Autodesk Inventor part; units mm, degrees
(part 5 of 7)
sketch "Dach z grawerem" plane through (0, 0, 2) normal (0, 0, 1) x (1, 0, 0)
  line L0 (-37.1273, -35.5639) -> (-39.2128, -35.5639) projected
  line L1 (-39.2128, -35.5639) -> (-40.0969, -34.6798) projected
  line L2 (-40.0969, -34.6798) -> (-40.0969, -31.5163) projected
  line L3 (-40.0969, -31.5163) -> (-39.2128, -30.6321) projected
  line L4 (-39.2128, -30.6321) -> (-37.1273, -30.6321) projected
  line L5 (-37.1273, -30.6321) -> (-36.2431, -31.5163) projected
  line L6 (-36.2431, -31.5163) -> (-36.2431, -34.6798) projected
  line L7 (-36.2431, -34.6798) -> (-37.1273, -35.5639) projected
  line L8 (-36.2431, -25.5358) -> (-40.0763, -25.5358) projected
  line L9 (-40.0763, -25.5358) -> (-40.7431, -24.2816) projected
  line L10 (-40.7431, -24.2816) -> (-36.2431, -24.2816) projected
  line L11 (-36.2431, -24.2816) -> (-36.2431, -25.5358) projected
  line L12 (-37.1273, -23.6971) -> (-39.2128, -23.6971) projected
  line L13 (-39.2128, -23.6971) -> (-40.0969, -22.8129) projected
  line L14 (-40.0969, -22.8129) -> (-40.0969, -19.6494) projected
  line L15 (-40.0969, -19.6494) -> (-39.2128, -18.7653) projected
  line L16 (-39.2128, -18.7653) -> (-37.1273, -18.7653) projected
  line L17 (-37.1273, -18.7653) -> (-36.2431, -19.6494) projected
  line L18 (-36.2431, -19.6494) -> (-36.2431, -22.8129) projected
  line L19 (-36.2431, -22.8129) -> (-37.1273, -23.6971) projected
  line L20 (4.635, -37.5613) -> (4.635, -40.3224) projected
  line L21 (4.635, -40.3224) -> (3.9927, -39.8015) projected
  line L22 (3.9927, -39.8015) -> (3.9927, -38.323) projected
  line L23 (3.9927, -38.323) -> (3.6441, -38.323) projected
  line L24 (3.6441, -38.323) -> (3.6441, -39.9973) projected
  line L25 (3.6441, -39.9973) -> (3.0527, -39.5176) projected
  line L26 (3.0527, -39.5176) -> (3.0527, -38.323) projected
  line L27 (3.0527, -38.323) -> (2.7042, -38.323) projected
  line L28 (2.7042, -38.323) -> (2.7042, -40.2441) projected
  line L29 (2.7042, -40.2441) -> (2.0619, -39.7193) projected
  line L30 (2.0619, -39.7193) -> (2.0619, -37.5613) projected
  line L31 (2.0619, -37.5613) -> (4.635, -37.5613) projected
  line L32 (4.635, -25.0404) -> (4.635, -27.8015) projected
  line L33 (4.635, -27.8015) -> (3.9927, -27.2806) projected
  line L34 (3.9927, -27.2806) -> (3.9927, -25.8022) projected
  line L35 (3.9927, -25.8022) -> (3.6421, -25.8022) projected
  line L36 (3.6421, -25.8022) -> (3.6421, -27.4764) projected
  line L37 (3.6421, -27.4764) -> (3.0508, -26.9967) projected
  line L38 (3.0508, -26.9967) -> (3.0508, -25.8022) projected
  line L39 (3.0508, -25.8022) -> (2.0795, -25.8022) projected
  line L40 (2.0795, -25.8022) -> (1.635, -25.0404) projected
  line L41 (1.635, -25.0404) -> (4.635, -25.0404) projected
  line L42 (3.8791, -22.7395) -> (3.2368, -22.7395) projected
  line L43 (3.2368, -22.7395) -> (3.2368, -22.1559) projected
  line L44 (3.2368, -22.1559) -> (3.8791, -22.1559) projected
  line L45 (3.8791, -22.1559) -> (3.8791, -22.7395) projected
  line L46 (5.0697, -18.5097) -> (2.6572, -18.5097) projected
  line L47 (2.6572, -18.5097) -> (2.0658, -17.9771) projected
  line L48 (2.0658, -17.9771) -> (2.0658, -16.2421) projected
  line L49 (2.0658, -16.2421) -> (2.6572, -15.7095) projected
  line L50 (2.6572, -15.7095) -> (4.6408, -15.7095) projected
  line L51 (2.7022, -16.4712) -> (2.7022, -17.7441) projected
  line L52 (2.7022, -17.7441) -> (4.6134, -17.7441) projected
  line L53 (4.6134, -17.7441) -> (5.0697, -18.5097) projected
  line L54 (4.635, -10.6279) -> (4.635, -12.8563) projected
  line L55 (2.7042, -12.778) -> (2.0619, -12.2532) projected
  line L56 (2.0619, -12.2532) -> (2.0619, -10.6259) projected
  line L57 (2.0619, -10.6259) -> (2.6454, -10.0952) projected
  line L58 (2.6454, -10.0952) -> (4.0416, -10.0952) projected
  line L59 (4.0416, -10.0952) -> (4.635, -10.6279) projected
  line L60 (2.7042, -4.949) -> (2.7042, -6.87) projected
  line L61 (2.7042, -6.87) -> (2.0619, -6.3452) projected
  line L62 (2.0619, -6.3452) -> (2.0619, -4.7179) projected
  line L63 (2.0619, -4.7179) -> (2.6454, -4.1873) projected
  line L64 (2.6454, -4.1873) -> (4.0416, -4.1873) projected
  line L65 (4.0514, -3.8191) -> (1.635, -3.8191) projected
  line L66 (1.635, -3.8191) -> (2.0795, -3.0535) projected
  line L67 (2.0795, -3.0535) -> (2.7786, -3.0535) projected
  line L68 (2.7786, -3.0535) -> (2.7786, -1.7806) projected
  line L69 (2.7786, -1.7806) -> (2.0619, -1.7806) projected
  line L70 (2.0619, -1.7806) -> (2.0658, -1.0189) projected
  line L71 (2.0658, -1.0189) -> (4.0514, -1.0189) projected
  line L72 (-58.6053, 8.1191) -> (-59.4082, 7.5578) projected
  line L73 (-59.4082, 7.5578) -> (-60.7496, 8.4879) projected
  line L74 (-60.7496, 8.4879) -> (-60.7496, 12.7634) projected
  line L75 (-60.7496, 12.7634) -> (-56.4611, 12.7634) projected
  line L76 (-59.4571, 13.4129) -> (-61.4611, 13.4129) projected
  line L77 (-61.4611, 13.4129) -> (-60.7137, 14.7445) projected
  line L78 (-60.7137, 14.7445) -> (-59.6889, 14.7445) projected
  line L79 (-59.6889, 14.7445) -> (-59.3592, 15.0676) projected
  line L80 (-59.3592, 15.0676) -> (-59.3592, 17.2347) projected
  line L81 (-59.3592, 17.2347) -> (-60.743, 17.2347) projected
  line L82 (-60.743, 17.2347) -> (-60.743, 18.5663) projected
  line L83 (-60.743, 18.5663) -> (-56.4611, 18.5663) projected
  line L84 (-56.4611, 18.5663) -> (-56.4611, 14.343) projected
  line L85 (-56.4611, 14.343) -> (-57.8057, 13.4129) projected
  line L86 (-57.8057, 13.4129) -> (-58.762, 14.095) projected
  line L87 (-58.762, 14.095) -> (-59.4571, 13.4129) projected
  line L88 (-56.4611, 29.8554) -> (-56.4611, 24.4344) projected
  line L89 (-56.4611, 24.4344) -> (-57.5218, 25.3515) projected
  line L90 (-57.5218, 25.3515) -> (-57.5218, 26.4807) projected
  line L91 (-57.5218, 26.4807) -> (-60.7137, 26.4807) projected
  line L92 (-60.7137, 26.4807) -> (-61.4611, 27.8123) projected
  line L93 (-61.4611, 27.8123) -> (-57.5218, 27.8123) projected
  line L94 (-57.5218, 27.8123) -> (-57.5218, 28.9416) projected
  line L95 (-57.5218, 28.9416) -> (-56.4611, 29.8554) projected
  line L96 (-75.6403, -50.5982) -> (-75.4415, -50.7741) projected
  line L97 (-75.4415, -50.7741) -> (-75.2314, -50.5982) projected
  line L98 (-75.2314, -50.5982) -> (-75.2314, -48.4484) projected
  line L99 (-75.2314, -48.4484) -> (-74.3267, -47.8041) projected
  line L100 (-74.3267, -47.8041) -> (-73.3854, -48.4689) projected
  line L101 (-73.3854, -48.4689) -> (-73.3854, -51.8113) projected
  line L102 (-73.3854, -51.8113) -> (-74.1279, -51.151) projected
  line L103 (-74.1279, -51.151) -> (-74.1279, -49.0149) projected
  line L104 (-74.1279, -49.0149) -> (-74.3267, -48.8367) projected
  line L105 (-74.3267, -48.8367) -> (-74.5368, -49.0149) projected
  line L106 (-74.5368, -49.0149) -> (-74.5368, -51.1648) projected
  line L107 (-75.6403, -41.3616) -> (-75.6403, -43.7787) projected
  line L108 (-75.6403, -43.7787) -> (-76.3874, -43.1184) projected
  line L109 (-76.3874, -43.1184) -> (-76.3874, -40.4112) projected
  line L110 (-76.3874, -40.4112) -> (-73.4082, -40.4112) projected
  line L111 (-72.8782, -41.3616) -> (-75.6403, -41.3616) projected
  line L112 (-73.3854, -39.4905) -> (-74.3267, -40.1553) projected
  line L113 (-74.3267, -40.1553) -> (-75.4141, -39.3854) projected
  line L114 (-75.4141, -39.3854) -> (-75.4141, -37.4229) projected
  line L115 (-75.4141, -37.4229) -> (-76.8854, -37.4229) projected
  line L116 (-76.8854, -37.4229) -> (-76.3622, -36.4725) projected
  line L117 (-76.3622, -36.4725) -> (-73.3854, -36.4725) projected
  line L118 (-73.3854, -36.4725) -> (-73.3854, -39.4905) projected
  line L119 (-74.5368, -28.9836) -> (-75.4438, -29.6302) projected
  line L120 (-75.4438, -29.6302) -> (-76.3828, -28.9653) projected
  line L121 (-76.3828, -28.9653) -> (-76.3828, -25.623) projected
  line L122 (-76.3828, -25.623) -> (-75.6403, -26.2764) projected
  line L123 (-75.6403, -26.2764) -> (-75.6403, -28.417) projected
  line L124 (-75.6403, -28.417) -> (-75.4415, -28.593) projected
  line L125 (-75.4415, -28.593) -> (-75.2314, -28.417) projected
  line L126 (-75.2314, -28.417) -> (-75.2314, -26.2672) projected
  line L127 (-75.2314, -26.2672) -> (-74.3267, -25.623) projected
  line L128 (-74.3267, -25.623) -> (-73.3854, -26.2878) projected
  line L129 (-73.3854, -26.2878) -> (-73.3854, -29.6302) projected
  line L130 (-73.3854, -29.6302) -> (-74.1279, -28.9699) projected
  line L131 (-74.1279, -28.9699) -> (-74.1279, -26.8338) projected
  line L132 (-74.1279, -26.8338) -> (-74.3267, -26.6556) projected
  line L133 (-74.3267, -26.6556) -> (-74.5368, -26.8338) projected
  line L134 (-74.5368, -26.8338) -> (-74.5368, -28.9836) projected
  line L135 (-75.6403, -19.1804) -> (-75.6403, -21.5975) projected
  line L136 (-75.6403, -21.5975) -> (-76.3874, -20.9373) projected
  line L137 (-76.3874, -20.9373) -> (-76.3874, -18.23) projected
  line L138 (-76.3874, -18.23) -> (-73.4082, -18.23) projected
  line L139 (-73.4082, -18.23) -> (-72.8782, -19.1804) projected
  line L140 (-72.8782, -19.1804) -> (-75.6403, -19.1804) projected
  line L141 (-73.3854, -17.3093) -> (-74.3267, -17.9742) projected
  line L142 (-74.3267, -17.9742) -> (-75.4141, -17.2042) projected
  line L143 (-75.4141, -17.2042) -> (-75.4141, -15.2418) projected
  line L144 (-75.4141, -15.2418) -> (-76.8854, -15.2418) projected
  line L145 (-76.8854, -15.2418) -> (-76.3622, -14.2914) projected
  line L146 (-62.0137, -37.4249) -> (-62.0137, -39.8107) projected
  line L147 (-62.0137, -39.8107) -> (-63.3037, -39.2171) projected
  line L148 (-63.3037, -39.2171) -> (-71.4886, -39.2171) projected
  line L149 (-71.4886, -39.2171) -> (-71.4886, -37.4934) projected
  line L150 (-71.4886, -37.4934) -> (-63.6576, -37.4934) projected
  line L151 (-63.6576, -37.4934) -> (-63.6576, -36.66) projected
  line L152 (-63.6576, -36.66) -> (-62.0137, -37.4249) projected
  line L153 (-69.8448, -24.845) -> (-69.8448, -28.7491) projected
  line L154 (-69.8448, -28.7491) -> (-71.4886, -27.9728) projected
  line L155 (-71.4886, -27.9728) -> (-71.4886, -23.1212) projected
  line L156 (-71.4886, -23.1212) -> (-63.5891, -23.1212) projected
  line L157 (-63.5891, -23.1212) -> (-63.0069, -22.4705) projected
  line L158 (-62.0137, -10.5642) -> (-62.0137, -12.95) projected
  line L159 (-62.0137, -12.95) -> (-63.3037, -12.3564) projected
  line L160 (-63.3037, -12.3564) -> (-71.7398, -12.3564) projected
  line L161 (-71.7398, -12.3564) -> (-64.7078, -7.0938) projected
  line L162 (-64.7078, -7.0938) -> (-69.8448, -7.0938) projected
  line L163 (-69.8448, -7.0938) -> (-69.8448, -9.4911) projected
  line L164 (-69.8448, -9.4911) -> (-71.4886, -8.7263) projected
  line L165 (-71.4886, -8.7263) -> (-71.4886, -5.8381) projected
  line L166 (-71.4886, -5.8381) -> (-70.0731, -6.4888) projected
  line L167 (-70.0731, -6.4888) -> (-63.8973, -6.4888) projected
  line L168 (-63.8973, -6.4888) -> (-63.0069, -5.8381) projected
  line L169 (-63.0069, -5.8381) -> (-61.7398, -7.0596) projected
  line L170 (-61.7398, -7.0596) -> (-68.0297, -11.7514) projected
  line L171 (-68.0297, -11.7514) -> (-63.6576, -11.7514) projected
  line L172 (-63.6576, -11.7514) -> (-63.6576, -9.7993) projected
  line L173 (-63.6576, -9.7993) -> (-62.0137, -10.5642) projected
  line L174 (-64.9704, -4.4454) -> (-69.0571, -4.4454) projected
  line L175 (-70.4727, -5.1075) -> (-71.7398, -3.8861) projected
  line L176 (-69.5252, -2.7331) -> (-66.7284, -2.7331) projected
  line L177 (-66.7284, -2.7331) -> (-66.7284, -0.2445) projected
  line L178 (-66.7284, -0.2445) -> (-71.4886, -0.2445) projected
  line L179 (-71.4886, -0.2445) -> (-71.4886, 1.4792) projected
  line L180 (-71.4886, 1.4792) -> (-63.5891, 1.4792) projected
  line L181 (-63.5891, 1.4792) -> (-63.0069, 2.1299) projected
  line L182 (-66.7284, 12.381) -> (-66.7284, 15.2692) projected
  line L183 (-66.7284, 15.2692) -> (-69.8448, 15.2692) projected
  line L184 (-69.8448, 15.2692) -> (-69.8448, 11.3651) projected
  line L185 (-69.8448, 11.3651) -> (-71.4886, 12.1413) projected
  line L186 (-71.4886, 12.1413) -> (-71.4886, 16.9929) projected
  line L187 (-63.6576, 15.2692) -> (-66.4772, 15.2692) projected
  line L188 (-66.4772, 15.2692) -> (-65.2101, 14.687) projected
  line L189 (-65.2101, 14.687) -> (-65.2101, 11.6733) projected
  line L190 (-65.2101, 11.6733) -> (-66.7284, 12.381) projected
  line L191 (-51.7783, 18.0076) -> (-51.3215, 17.568) projected
  line L192 (-51.3215, 17.568) -> (-50.9232, 17.2377) projected
  line L193 (-50.9232, 17.2377) -> (-50.2693, 16.6848) projected
  line L194 (-50.2693, 16.6848) -> (-49.9951, 16.4297) projected
  line L195 (-49.9951, 16.4297) -> (-50.165, 16.3033) projected
  line L196 (-50.165, 16.3033) -> (-50.5, 16.1442) projected
  line L197 (-50.5, 16.1442) -> (-51.1005, 15.9331) projected
  line L198 (-51.1005, 15.9331) -> (-51.8054, 15.7225) projected
  line L199 (-51.8054, 15.7225) -> (-52.454, 15.5646) projected
  line L200 (-52.454, 15.5646) -> (-52.9492, 15.4449) projected
  line L201 (-52.9492, 15.4449) -> (-53.3651, 15.3143) projected
  line L202 (-53.3651, 15.3143) -> (-53.7749, 15.1819) projected
  line L203 (-53.7749, 15.1819) -> (-53.8063, 15.279) projected
  line L204 (-53.8063, 15.279) -> (-53.7947, 15.5136) projected
  line L205 (-53.7947, 15.5136) -> (-53.3572, 19.0396) projected
  line L206 (-53.3572, 19.0396) -> (-53.3518, 19.1652) projected
  line L207 (-53.3518, 19.1652) -> (-53.3854, 19.2823) projected
  line L208 (-53.3854, 19.2823) -> (-53.6091, 19.5839) projected
  line L209 (-53.6091, 19.5839) -> (-53.7889, 19.8131) projected
  line L210 (-53.7889, 19.8131) -> (-53.8265, 19.9093) projected
  line L211 (-53.8265, 19.9093) -> (-53.8193, 19.9314) projected
  line L212 (-53.8193, 19.9314) -> (-53.8756, 19.9801) projected
  line L213 (-53.8756, 19.9801) -> (-53.9256, 20.0367) projected
  line L214 (-53.9256, 20.0367) -> (-53.8118, 20.0504) projected
  line L215 (-53.8118, 20.0504) -> (-53.7148, 20.0243) projected
  line L216 (-53.7148, 20.0243) -> (-53.5909, 19.9446) projected
  line L217 (-53.5909, 19.9446) -> (-53.2491, 19.6107) projected
  line L218 (-53.2491, 19.6107) -> (-51.7783, 18.0076) projected
  line L219 (-50.3026, 20.472) -> (-51.1482, 20.6427) projected
  line L220 (-51.1482, 20.6427) -> (-52.0028, 20.7487) projected
  line L221 (-52.0028, 20.7487) -> (-52.9213, 20.8512) projected
  line L222 (-52.9213, 20.8512) -> (-53.1471, 20.912) projected
  line L223 (-53.1471, 20.912) -> (-53.2788, 20.9937) projected
  line L224 (-53.2788, 20.9937) -> (-53.3233, 21.0901) projected
  line L225 (-53.3233, 21.0901) -> (-53.2667, 21.1656) projected
  line L226 (-53.2667, 21.1656) -> (-53.1401, 21.2025) projected
  line L227 (-53.1401, 21.2025) -> (-52.9747, 21.183) projected
  line L228 (-52.9747, 21.183) -> (-52.2132, 21.067) projected
  line L229 (-52.2132, 21.067) -> (-51.2901, 20.9848) projected
  line L230 (-51.2901, 20.9848) -> (-50.8379, 20.9204) projected
  line L231 (-50.8379, 20.9204) -> (-50.4854, 20.8414) projected
  line L232 (-50.4854, 20.8414) -> (-49.7014, 20.623) projected
  line L233 (-49.7014, 20.623) -> (-49.3537, 20.4935) projected
  line L234 (-49.3537, 20.4935) -> (-49.1396, 20.3844) projected
  line L235 (-49.1396, 20.3844) -> (-49.029, 20.3131) projected
  line L236 (-49.029, 20.3131) -> (-48.946, 20.2928) projected
  line L237 (-48.946, 20.2928) -> (-48.8521, 20.3267) projected
  line L238 (-48.8521, 20.3267) -> (-48.7091, 20.418) projected
  line L239 (-48.7091, 20.418) -> (-48.4766, 20.5502) projected
  line L240 (-48.4766, 20.5502) -> (-48.2708, 20.6349) projected
  line L241 (-48.2708, 20.6349) -> (-48.1208, 20.6423) projected
  line L242 (-48.1208, 20.6423) -> (-48.0943, 20.6035) projected
  line L243 (-48.0943, 20.6035) -> (-48.0878, 20.5284) projected
  line L244 (-48.0878, 20.5284) -> (-48.1306, 20.4095) projected
  line L245 (-48.1306, 20.4095) -> (-48.2579, 20.3385) projected
  line L246 (-48.2579, 20.3385) -> (-48.4307, 20.2573) projected
  line L247 (-48.4307, 20.2573) -> (-48.6019, 20.108) projected
  line L248 (-48.6019, 20.108) -> (-48.7427, 19.9228) projected
  line L249 (-48.7427, 19.9228) -> (-48.8248, 19.734) projected
  line L250 (-48.8248, 19.734) -> (-48.9463, 19.3465) projected
  line L251 (-48.9463, 19.3465) -> (-49.0427, 19.0452) projected
  line L252 (-49.0427, 19.0452) -> (-49.1406, 18.3947) projected
  line L253 (-49.1406, 18.3947) -> (-49.1671, 17.9451) projected
  line L254 (-49.1671, 17.9451) -> (-49.1087, 17.5479) projected
  line L255 (-49.1087, 17.5479) -> (-48.9698, 17.0753) projected
  line L256 (-48.9698, 17.0753) -> (-48.8063, 16.633) projected
  line L257 (-48.8063, 16.633) -> (-48.6386, 16.2701) projected
  line L258 (-48.6386, 16.2701) -> (-48.4868, 16.0355) projected
  line L259 (-48.4868, 16.0355) -> (-48.3041, 15.8443) projected
  line L260 (-48.3041, 15.8443) -> (-47.4502, 15.8903) projected
  line L261 (-47.4502, 15.8903) -> (-46.7506, 15.9386) projected
  line L262 (-46.7506, 15.9386) -> (-46.2786, 15.9985) projected
  line L263 (-46.2786, 15.9985) -> (-45.9672, 16.1121) projected
  line L264 (-45.9672, 16.1121) -> (-45.6158, 16.3115) projected
  line L265 (-45.6158, 16.3115) -> (-45.2403, 16.5876) projected
  line L266 (-45.2403, 16.5876) -> (-44.8566, 16.9311) projected
  line L267 (-44.8566, 16.9311) -> (-44.5098, 17.3449) projected
  line L268 (-44.5098, 17.3449) -> (-44.1286, 17.9107) projected
  line L269 (-44.1286, 17.9107) -> (-43.7936, 18.5005) projected
  line L270 (-43.7936, 18.5005) -> (-43.5854, 18.9863) projected
  line L271 (-43.5854, 18.9863) -> (-43.4569, 19.3738) projected
  line L272 (-43.4569, 19.3738) -> (-43.3767, 19.7818) projected
  line L273 (-43.3767, 19.7818) -> (-43.3327, 20.4387) projected
  line L274 (-43.3327, 20.4387) -> (-43.3367, 20.7012) projected
  line L275 (-43.3367, 20.7012) -> (-43.3713, 20.9143) projected
  line L276 (-43.3713, 20.9143) -> (-43.4509, 21.1367) projected
  line L277 (-43.4509, 21.1367) -> (-43.5897, 21.4275) projected
  line L278 (-43.5897, 21.4275) -> (-43.7987, 21.8117) projected
  line L279 (-43.7987, 21.8117) -> (-43.9901, 22.0986) projected
  line L280 (-43.9901, 22.0986) -> (-44.1568, 22.2781) projected
  line L281 (-44.1568, 22.2781) -> (-44.2916, 22.3405) projected
  line L282 (-44.2916, 22.3405) -> (-44.4801, 22.4154) projected
  line L283 (-44.4801, 22.4154) -> (-44.8057, 22.5966) projected
  line L284 (-44.8057, 22.5966) -> (-45.852, 23.1688) projected
  line L285 (-45.852, 23.1688) -> (-46.8407, 23.6137) projected
  line L286 (-46.8407, 23.6137) -> (-47.862, 24.0482) projected
  line L287 (-47.862, 24.0482) -> (-48.7354, 24.4045) projected
  line L288 (-48.7354, 24.4045) -> (-49.7216, 24.8106) projected
  line L289 (-49.7216, 24.8106) -> (-50.9261, 25.3244) projected
  line L290 (-50.9261, 25.3244) -> (-51.358, 25.4849) projected
  line L291 (-51.358, 25.4849) -> (-51.5813, 25.5448) projected
  line L292 (-51.5813, 25.5448) -> (-52.0252, 25.6948) projected
  arc A0 (-52.0652, 26.0877) -> (-52.0252, 25.6948) centre (-51.9558, 25.9004) ccw projected
  line L293 (-52.0652, 26.0877) -> (-51.3968, 25.8193) projected
  line L294 (-51.3968, 25.8193) -> (-49.9175, 25.2277) projected
  line L295 (-49.9175, 25.2277) -> (-48.6002, 24.6932) projected
  line L296 (-48.6002, 24.6932) -> (-47.7937, 24.3584) projected
  line L297 (-47.7937, 24.3584) -> (-47.1564, 24.0454) projected
  line L298 (-47.1564, 24.0454) -> (-47.0155, 23.9884) projected
  line L299 (-47.0155, 23.9884) -> (-46.6961, 23.8893) projected
  line L300 (-46.6961, 23.8893) -> (-46.252, 23.7057) projected
  line L301 (-46.252, 23.7057) -> (-45.2196, 23.1839) projected
  line L302 (-45.2196, 23.1839) -> (-44.3747, 22.736) projected
  line L303 (-44.3747, 22.736) -> (-44.0527, 22.5468) projected
  line L304 (-44.0527, 22.5468) -> (-43.7204, 22.2677) projected
  line L305 (-43.7204, 22.2677) -> (-43.3928, 21.709) projected
  line L306 (-43.3928, 21.709) -> (-43.0973, 21.0657) projected
  line L307 (-43.0973, 21.0657) -> (-43.0417, 20.7944) projected
  line L308 (-43.0417, 20.7944) -> (-43.0222, 20.4472) projected
  line L309 (-43.0222, 20.4472) -> (-43.0398, 20.0564) projected
  line L310 (-43.0398, 20.0564) -> (-43.0959, 19.6546) projected
  line L311 (-43.0959, 19.6546) -> (-43.2066, 19.1823) projected
  line L312 (-43.2066, 19.1823) -> (-43.3617, 18.6996) projected
  line L313 (-43.3617, 18.6996) -> (-43.523, 18.3069) projected
  line L314 (-43.523, 18.3069) -> (-43.6525, 18.1046) projected
  line L315 (-43.6525, 18.1046) -> (-43.9366, 17.6189) projected
  line L316 (-43.9366, 17.6189) -> (-44.1239, 17.307) projected
  line L317 (-44.1239, 17.307) -> (-44.3421, 17.0243) projected
  line L318 (-44.3421, 17.0243) -> (-44.6358, 16.7208) projected
  line L319 (-44.6358, 16.7208) -> (-45.0495, 16.3463) projected
  line L320 (-45.0495, 16.3463) -> (-45.3942, 16.0747) projected
  line L321 (-45.3942, 16.0747) -> (-45.742, 15.8693) projected
  line L322 (-45.742, 15.8693) -> (-46.0987, 15.7274) projected
  line L323 (-46.0987, 15.7274) -> (-46.4705, 15.6464) projected
  line L324 (-46.4705, 15.6464) -> (-47.0347, 15.6011) projected
  line L325 (-47.0347, 15.6011) -> (-47.6755, 15.5878) projected
  line L326 (-47.6755, 15.5878) -> (-48.2288, 15.6059) projected
  line L327 (-48.2288, 15.6059) -> (-48.5307, 15.6547) projected
  line L328 (-48.5307, 15.6547) -> (-48.6845, 15.7938) projected
  line L329 (-48.6845, 15.7938) -> (-48.8538, 16.0229) projected
  line L330 (-48.8538, 16.0229) -> (-49.1485, 16.652) projected
  line L331 (-49.1485, 16.652) -> (-49.2499, 16.9453) projected
  line L332 (-49.2499, 16.9453) -> (-49.2588, 17.0688) projected
  line L333 (-49.2588, 17.0688) -> (-49.3285, 17.2666) projected
  line L334 (-49.3285, 17.2666) -> (-49.4065, 17.4636) projected
  line L335 (-49.4065, 17.4636) -> (-49.4566, 17.6925) projected
  line L336 (-49.4566, 17.6925) -> (-49.4737, 18.2364) projected
  line L337 (-49.4737, 18.2364) -> (-49.3806, 18.8791) projected
  line L338 (-49.3806, 18.8791) -> (-49.1781, 19.6014) projected
  line L339 (-49.1781, 19.6014) -> (-49.1227, 19.7813) projected
  line L340 (-49.1227, 19.7813) -> (-49.1099, 19.8939) projected
  line L341 (-49.1099, 19.8939) -> (-49.1448, 19.9803) projected
  line L342 (-49.1448, 19.9803) -> (-49.2326, 20.0814) projected
  line L343 (-49.2326, 20.0814) -> (-49.376, 20.1738) projected
  line L344 (-49.376, 20.1738) -> (-49.6145, 20.2728) projected
  line L345 (-49.6145, 20.2728) -> (-50.3026, 20.472) projected
  line L346 (-45.9525, 18.1279) -> (-45.9298, 18.1594) projected
  line L347 (-45.9298, 18.1594) -> (-45.8933, 18.1577) projected
  line L348 (-45.8933, 18.1577) -> (-45.7764, 18.0496) projected
  line L349 (-45.7764, 18.0496) -> (-45.6289, 17.8868) projected
  line L350 (-45.6289, 17.8868) -> (-45.7776, 17.7533) projected
  line L351 (-45.7776, 17.7533) -> (-45.8998, 17.6649) projected
  line L352 (-45.8998, 17.6649) -> (-46.0012, 17.6307) projected
  line L353 (-46.0012, 17.6307) -> (-46.0985, 17.6494) projected
  line L354 (-46.0985, 17.6494) -> (-46.2081, 17.7197) projected
  line L355 (-46.2081, 17.7197) -> (-46.2717, 17.7714) projected
  line L356 (-46.2717, 17.7714) -> (-46.2942, 17.8189) projected
  line L357 (-46.2942, 17.8189) -> (-46.2213, 17.9597) projected
  line L358 (-46.2213, 17.9597) -> (-46.1283, 18.0616) projected
  line L359 (-46.1283, 18.0616) -> (-46.0515, 18.079) projected
  line L360 (-46.0515, 18.079) -> (-45.9994, 18.0796) projected
  line L361 (-45.9994, 18.0796) -> (-45.9525, 18.1279) projected
  line L362 (-69.274, 4.3103) -> (-71.7512, 6.2623) projected
  line L363 (-71.7512, 6.2623) -> (-71.4886, 6.6505) projected
  line L364 (-71.4886, 6.6505) -> (-71.4886, 8.0888) projected
  line L365 (-71.4886, 8.0888) -> (-63.5891, 9.9952) projected
  line L366 (-63.5891, 9.9952) -> (-63.0069, 10.6459) projected
  line L367 (-64.8334, -16.8769) -> (-64.8334, -19.5368) projected
  line L368 (-69.0115, -20.7925) -> (-71.7512, -18.6349) projected
  line L369 (-71.7512, -18.6349) -> (-71.4544, -18.1441) projected
  line L370 (-69.8448, -32.0253) -> (-69.8448, -35.9409) projected
  line L371 (-69.8448, -35.9409) -> (-71.4886, -35.1646) projected
  line L372 (-71.4886, -35.1646) -> (-71.4886, -30.3016) projected
  line L373 (-71.4886, -30.3016) -> (-63.6576, -30.3016) projected
  line L374 (-63.6576, -30.3016) -> (-63.6576, -29.4683) projected
  line L375 (-63.6576, -29.4683) -> (-62.0137, -30.2331) projected
  line L376 (-71.7512, -45.5299) -> (-71.4658, -45.1418) projected
  line L377 (-61.7398, -43.0413) -> (-62.0137, -43.4409) projected
  line L378 (-62.0137, -43.4409) -> (-62.0137, -46.1007) projected
  line L379 (-62.0137, -46.1007) -> (-62.3905, -45.918) projected
  line L380 (-64.7078, -50.1874) -> (-69.8448, -50.1874) projected
  line L381 (-69.8448, -50.1874) -> (-69.8448, -52.5847) projected
  line L382 (-69.8448, -52.5847) -> (-71.4886, -51.8199) projected
  line L383 (-71.4886, -51.8199) -> (-71.4886, -48.9317) projected
  line L384 (-71.4886, -48.9317) -> (-70.0731, -49.5824) projected
  line L385 (-70.0731, -49.5824) -> (-63.8973, -49.5824) projected
  line L386 (-63.8973, -49.5824) -> (-63.0069, -48.9317) projected
  line L387 (-72.8782, -25.1752) -> (-75.6928, -25.1752) projected
  line L388 (-75.6928, -25.1752) -> (-76.3828, -24.5058) projected
  line L389 (-76.3828, -24.5058) -> (-76.3828, -22.3309) projected
  line L390 (-76.3828, -22.3309) -> (-75.6928, -21.6615) projected
  line L391 (-75.6928, -21.6615) -> (-73.3785, -21.6615) projected
  line L392 (-73.3785, -21.6615) -> (-73.3854, -22.6119) projected
  line L393 (-73.3854, -22.6119) -> (-75.6403, -22.6119) projected
  line L394 (-75.6403, -22.6119) -> (-75.6403, -24.2202) projected
  line L395 (-75.6403, -24.2202) -> (-73.4082, -24.2202) projected
  line L396 (-73.4082, -24.2202) -> (-72.8782, -25.1752) projected
  line L397 (-72.8782, -33.4843) -> (-75.6928, -33.4843) projected
  line L398 (-75.6928, -33.4843) -> (-76.3828, -32.8149) projected
  line L399 (-76.3828, -32.8149) -> (-76.3828, -30.6399) projected
  line L400 (-76.3828, -30.6399) -> (-75.6928, -29.9706) projected
  line L401 (-75.6928, -29.9706) -> (-73.3785, -29.9706) projected
  line L402 (-75.6403, -30.921) -> (-75.6403, -32.5293) projected
  line L403 (-75.6403, -32.5293) -> (-73.4082, -32.5293) projected
  line L404 (-73.4082, -32.5293) -> (-72.8782, -33.4843) projected
  line L405 (-72.8782, -47.3563) -> (-75.6928, -47.3563) projected
  line L406 (-75.6928, -47.3563) -> (-76.3828, -46.6869) projected
  line L407 (-76.3828, -46.6869) -> (-76.3828, -44.512) projected
  line L408 (-76.3828, -44.512) -> (-75.6928, -43.8426) projected
  line L409 (-75.6928, -43.8426) -> (-73.3785, -43.8426) projected
  line L410 (-73.3785, -43.8426) -> (-73.3854, -44.793) projected
  line L411 (-73.3854, -44.793) -> (-75.6403, -44.793) projected
  line L412 (-75.6403, -44.793) -> (-75.6403, -46.4014) projected
  line L413 (-75.6403, -46.4014) -> (-73.4082, -46.4014) projected
  line L414 (-73.4082, -46.4014) -> (-72.8782, -47.3563) projected
  line L415 (-72.8782, -55.6654) -> (-75.6928, -55.6654) projected
  line L416 (-75.6928, -55.6654) -> (-76.3828, -54.996) projected
  line L417 (-76.3828, -54.996) -> (-76.3828, -52.8211) projected
  line L418 (-76.3828, -52.8211) -> (-75.6928, -52.1517) projected
  line L419 (-75.6928, -52.1517) -> (-73.3785, -52.1517) projected
  line L420 (-59.7574, 19.1896) -> (-60.743, 20.1263) projected
  line L421 (-60.743, 20.1263) -> (-60.743, 23.1746) projected
  line L422 (-60.743, 23.1746) -> (-59.7607, 24.108) projected
  line L423 (-59.7607, 24.108) -> (-56.4513, 24.108) projected
  line L424 (-56.4513, 24.108) -> (-56.4611, 22.7764) projected
  line L425 (-56.4611, 22.7764) -> (-59.6823, 22.7764) projected
  line L426 (-59.6823, 22.7764) -> (-59.6823, 20.5277) projected
  line L427 (-57.4467, 1.7484) -> (-59.7574, 1.7484) projected
  line L428 (-59.7574, 1.7484) -> (-60.743, 2.6851) projected
  line L429 (-60.743, 2.6851) -> (-60.743, 6.0271) projected
  line L430 (-60.743, 6.0271) -> (-59.7607, 6.9605) projected
  line L431 (-59.7607, 6.9605) -> (-57.4434, 6.9605) projected
  line L432 (-57.4434, 6.9605) -> (-56.4611, 6.0271) projected
  line L433 (-56.4611, 6.0271) -> (-56.4611, 2.6851) projected
  line L434 (-56.4611, 2.6851) -> (-57.4467, 1.7484) projected
  line L435 (4.635, -0.6586) -> (2.0619, -0.6586) projected
  line L436 (2.0619, -0.6586) -> (2.0619, 0.1032) projected
  line L437 (2.0619, 0.1032) -> (3.0508, 0.1032) projected
  line L438 (3.0508, 0.1032) -> (3.0508, 1.3525) projected
  line L439 (3.0508, 1.3525) -> (2.0795, 1.3525) projected
  line L440 (2.0795, 1.3525) -> (1.635, 2.1143) projected
  line L441 (4.635, 1.3525) -> (3.6421, 1.3525) projected
  line L442 (3.6421, 1.3525) -> (3.6421, 0.1032) projected
  line L443 (3.6421, 0.1032) -> (4.635, 0.1032) projected
  line L444 (4.635, 0.1032) -> (4.635, -0.6586) projected
  line L445 (3.225, -8.5091) -> (2.4946, -7.8354) projected
  line L446 (2.4946, -7.8354) -> (2.0619, -7.8354) projected
  line L447 (2.0619, -7.8354) -> (2.0658, -7.0737) projected
  line L448 (2.0658, -7.0737) -> (4.635, -7.0737) projected
  line L449 (2.7042, -13.7434) -> (2.7042, -15.6644) projected
  line L450 (2.7042, -15.6644) -> (2.0619, -15.1396) projected
  line L451 (2.0619, -15.1396) -> (2.0619, -12.9817) projected
  line L452 (2.0619, -12.9817) -> (4.6134, -12.9817) projected
  line L453 (4.6134, -12.9817) -> (5.0697, -13.7434) projected
  line L454 (5.0697, -13.7434) -> (2.7042, -13.7434) projected
  line L455 (3.3484, -21.5019) -> (2.8667, -21.8211) projected
  line L456 (2.8667, -21.8211) -> (2.0619, -21.2924) projected
  line L457 (2.0619, -21.2924) -> (2.0619, -18.8583) projected
  line L458 (2.0619, -18.8583) -> (4.635, -18.8583) projected
  line L459 (2.71, -22.7395) -> (2.0736, -22.7395) projected
  line L460 (2.0736, -22.7395) -> (2.0736, -22.1559) projected
  line L461 (2.0736, -22.1559) -> (2.71, -22.1559) projected
  line L462 (2.71, -22.1559) -> (2.71, -22.7395) projected
  line L463 (2.6572, -30.8857) -> (2.0658, -30.3531) projected
  line L464 (2.0658, -30.3531) -> (2.0658, -28.4516) projected
  line L465 (2.0658, -28.4516) -> (2.6572, -27.919) projected
  line L466 (2.6572, -27.919) -> (4.0436, -27.919) projected
  line L467 (4.0436, -27.919) -> (4.635, -28.4516) projected
  line L468 (2.8961, -33.216) -> (2.8961, -31.9882) projected
  line L469 (2.8961, -31.9882) -> (2.0658, -31.9882) projected
  line L470 (2.0658, -31.9882) -> (2.0658, -31.2264) projected
  line L471 (2.0658, -31.2264) -> (4.635, -31.2264) projected
  line L472 (4.635, -35.0567) -> (4.635, -37.2852) projected
  line L473 (4.635, -37.2852) -> (3.9927, -36.7643) projected
  line L474 (3.9927, -36.7643) -> (3.9927, -35.2858) projected
  line L475 (3.9927, -35.2858) -> (2.7042, -35.2858) projected
  line L476 (2.7042, -35.2858) -> (2.7042, -36.4451) projected
  line L477 (2.7042, -36.4451) -> (3.0527, -36.4451) projected
  line L478 (3.0527, -36.4451) -> (3.0527, -36.0045) projected
  line L479 (3.0527, -36.0045) -> (3.6441, -35.5267) projected
  line L480 (3.6441, -35.5267) -> (3.6441, -37.2069) projected
  line L481 (3.6441, -37.2069) -> (2.6474, -37.2069) projected
  line L482 (2.6474, -37.2069) -> (2.0619, -36.6821) projected
  line L483 (2.0619, -36.6821) -> (2.0619, -35.0567) projected
  line L484 (2.0619, -35.0567) -> (2.6454, -34.5241) projected
  line L485 (2.6454, -34.5241) -> (4.0416, -34.5241) projected
  line L486 (4.0416, -34.5241) -> (4.635, -35.0567) projected
  line L487 (-38.9396, -7.1334) -> (-40.0969, -7.1334) projected
  line L488 (-40.0969, -7.1334) -> (-40.0969, -5.8792) projected
  line L489 (-40.0969, -5.8792) -> (-39.1511, -5.8792) projected
  line L490 (-39.1511, -5.8792) -> (-38.8515, -5.5708) projected
  line L491 (-38.8515, -5.5708) -> (-38.8515, -3.5117) projected
  line L492 (-38.8515, -3.5117) -> (-40.0705, -3.5117) projected
  line L493 (-40.0705, -3.5117) -> (-40.7431, -2.2574) projected
  line L494 (-40.7431, -2.2574) -> (-36.2431, -2.2574) projected
  line L495 (-36.2431, -2.2574) -> (-36.2431, -6.2522) projected
  line L496 (-38.3139, -6.4872) -> (-38.9396, -7.1334) projected
  line L497 (-39.2128, -12.685) -> (-40.0969, -11.8008) projected
  line L498 (-40.0969, -11.8008) -> (-40.0969, -8.6373) projected
  line L499 (-40.0969, -8.6373) -> (-39.2128, -7.7532) projected
  line L500 (-39.2128, -7.7532) -> (-37.1273, -7.7532) projected
  line L501 (-38.1729, -17.6638) -> (-38.8955, -18.1954) projected
  line L502 (-38.8955, -18.1954) -> (-40.1028, -17.3142) projected
  line L503 (-40.1028, -17.3142) -> (-40.1028, -13.2695) projected
  line L504 (-40.1028, -13.2695) -> (-36.2431, -13.2695) projected
  line L505 (-36.2431, -13.2695) -> (-36.2431, -17.3142) projected
  line L506 (-36.2431, -17.3142) -> (-37.4504, -18.1954) projected
  line L507 (-37.4504, -18.1954) -> (-38.1729, -17.6638) projected
  line L508 (-39.1423, -27.3394) -> (-39.1423, -30.5411) projected
  line L509 (-39.1423, -30.5411) -> (-40.1028, -29.6687) projected
  line L510 (-40.1028, -29.6687) -> (-40.1028, -26.0851) projected
  line L511 (-40.1028, -26.0851) -> (-36.2725, -26.0851) projected
  line L512 (-36.2725, -26.0851) -> (-35.591, -27.3394) projected
  line L513 (-35.591, -27.3394) -> (-39.1423, -27.3394) projected
  circle A1 centre (-9.75, -51.55) radius 1.5 projected
  circle A2 centre (3.25, -51.55) radius 1.5 projected
  circle A3 centre (3.25, -45.05) radius 1.5 projected
  circle A4 centre (3.25, 6.65) radius 1.5 projected
  circle A5 centre (3.25, 13.15) radius 1.5 projected
  circle A6 centre (-9.75, 13.15) radius 1.5 projected
  circle A7 centre (-67.4121, -60.2) radius 1.5 projected
  circle A8 centre (-74.1621, -60.2) radius 1.5 projected
  circle A9 centre (-67.4121, 21.8) radius 1.5 projected
  circle A10 centre (-74.1621, 21.8) radius 1.5 projected
  arc A11 (-34.5609, -6.5715) -> (-34.319, -6.1433) centre (-34.819, -6.1433) ccw projected
  line L514 (-34.319, -6.1433) -> (-34.319, 1.7) projected
  arc A12 (-33.819, 2.2) -> (-34.319, 1.7) centre (-33.819, 1.7) ccw projected
  line L515 (-33.819, 2.2) -> (-31.9232, 2.2) projected
  arc A13 (-31.9232, 2.2) -> (-31.4585, 2.8843) centre (-31.9232, 2.7) ccw projected
  arc A14 (-23.3621, 2.3219) -> (-31.4585, 2.8843) centre (-27.2755, 4.5435) ccw projected
  arc A15 (-23.3621, 2.3219) -> (-22.9273, 1.575) centre (-22.9273, 2.075) ccw projected
  line L516 (-22.9273, 1.575) -> (-21.369, 1.575) projected
  arc A16 (-20.869, 1.075) -> (-21.369, 1.575) centre (-21.369, 1.075) ccw projected
  line L517 (-20.869, 1.075) -> (-20.869, -6) projected
  arc A17 (-20.869, -6) -> (-20.369, -6.5) centre (-20.369, -6) ccw projected
  line L518 (-20.369, -6.5) -> (-17.8027, -6.5) projected
  line L519 (-17.8027, -6.5) -> (-17.8027, -31.5) projected
  line L520 (-17.8027, -31.5) -> (-22.519, -31.5) projected
  arc A18 (-22.519, -31.5) -> (-23.019, -32) centre (-22.519, -32) ccw projected
  line L521 (-23.019, -32) -> (-23.019, -39.025) projected
  arc A19 (-23.519, -39.525) -> (-23.019, -39.025) centre (-23.519, -39.025) ccw projected
  line L522 (-23.519, -39.525) -> (-26.644, -39.525) projected
  arc A20 (-26.644, -39.525) -> (-27.144, -40.025) centre (-26.644, -40.025) ccw projected
  line L523 (-27.144, -40.025) -> (-27.144, -47.7) projected
  line L524 (-27.144, -47.7) -> (-32.144, -47.7) projected
  line L525 (-32.144, -47.7) -> (-32.144, -38.225) projected
  line L526 (-32.144, -38.225) -> (-28.019, -38.225) projected
  arc A21 (-28.019, -38.225) -> (-27.519, -37.725) centre (-28.019, -37.725) ccw projected
  line L527 (-27.519, -37.725) -> (-27.519, -32) projected
  arc A22 (-27.519, -32) -> (-28.019, -31.5) centre (-28.019, -32) ccw projected
  line L528 (-28.019, -31.5) -> (-34.8027, -31.5) projected
  line L529 (-34.8027, -31.5) -> (-34.8027, -6.9997) projected
  arc A23 (-34.5609, -6.5715) -> (-34.8027, -6.9997) centre (-34.3027, -6.9997) ccw projected
  arc A24 (-41.8371, -69.2) -> (-41.3371, -68.7) centre (-41.8371, -68.7) ccw projected
  line L530 (-41.3371, -68.7) -> (-41.3371, -49.7) projected
  line L531 (-41.3371, -49.7) -> (-13, -49.7) projected
  line L532 (-13, -49.7) -> (-13, -55.4) projected
  line L533 (-13, -55.4) -> (6.3, -55.4) projected
  line L534 (6.3, -55.4) -> (6.3, 17) projected
  line L535 (6.3, 17) -> (-13, 17) projected
  line L536 (-13, 17) -> (-13, 11.3) projected
  line L537 (-13, 11.3) -> (-41.3371, 11.3) projected
  line L538 (-41.3371, 11.3) -> (-41.3371, 30.3) projected
  arc A25 (-41.3371, 30.3) -> (-41.8371, 30.8) centre (-41.8371, 30.3) ccw projected
  line L539 (-41.8371, 30.8) -> (-78.3805, 30.8) projected
  line L540 (-78.3805, 30.8) -> (-78.3805, -69.2) projected
  line L541 (-78.3805, -69.2) -> (-41.8371, -69.2) projected
  line L542 (-56.7398, -38.1) -> (-56.7398, -0.3) projected
  line L543 (-56.2398, 0.2) -> (-42.0344, 0.2) projected
  line L544 (-41.5344, -0.3) -> (-41.5344, -38.1) projected
  line L545 (-42.0344, -38.6) -> (-56.2398, -38.6) projected
  line L546 (-15.3027, 0.2) -> (-1.0973, 0.2) projected
  line L547 (-0.5973, -0.3) -> (-0.5973, -38.1) projected
  line L548 (-1.0973, -38.6) -> (-15.3027, -38.6) projected
  line L549 (-15.8027, -38.1) -> (-15.8027, -0.3) projected
  arc A26 (-44.4926, 3.775) -> (-43.9933, 4.2482) centre (-44.4926, 4.275) ccw projected
  line L550 (-44.4926, 3.775) -> (-49.494, 3.775) projected
  arc A27 (-49.994, 4.275) -> (-49.494, 3.775) centre (-49.494, 4.275) ccw projected
  line L551 (-49.994, 4.275) -> (-49.994, 9.275) projected
  arc A28 (-49.494, 9.775) -> (-49.994, 9.275) centre (-49.494, 9.275) ccw projected
  line L552 (-49.494, 9.775) -> (-44.494, 9.775) projected
  arc A29 (-43.994, 9.275) -> (-44.494, 9.775) centre (-44.494, 9.275) ccw projected
  line L553 (-43.994, 9.275) -> (-43.994, 8.1787) projected
  arc A30 (-43.994, 8.1787) -> (-43.494, 7.6787) centre (-43.494, 8.1787) ccw projected
  line L554 (-43.494, 7.6787) -> (-38.269, 7.6787) projected
  arc A31 (-37.769, 7.1787) -> (-38.269, 7.6787) centre (-38.269, 7.1787) ccw projected
  line L555 (-37.769, 7.1787) -> (-37.769, 5.2213) projected
  arc A32 (-38.269, 4.7213) -> (-37.769, 5.2213) centre (-38.269, 5.2213) ccw projected
  line L556 (-38.269, 4.7213) -> (-43.494, 4.7213) projected
  arc A33 (-43.494, 4.7213) -> (-43.9933, 4.2482) centre (-43.494, 4.2213) ccw projected
  line L557 (-13.5155, 5.8092) -> (-8.3155, 5.8092) projected
  line L558 (-8.3155, 5.8092) -> (-8.3155, 0.6092) projected
  line L559 (-8.3155, 0.6092) -> (-13.5155, 0.6092) projected
  line L560 (-13.5155, 0.6092) -> (-13.5155, 5.8092) projected
  line L561 (-21.4873, -42.1072) -> (-16.2873, -42.1072) projected
  line L562 (-16.2873, -42.1072) -> (-16.2873, -47.3072) projected
  line L563 (-16.2873, -47.3072) -> (-21.4873, -47.3072) projected
  line L564 (-21.4873, -47.3072) -> (-21.4873, -42.1072) projected
  circle A34 centre (-17.024, 4.925) radius 1 projected
  line L565 (-37.1977, -5.5796) -> (-37.1977, -3.5117) projected
  line L566 (-37.1977, -3.5117) -> (-37.8763, -3.5117) projected
  line L567 (-37.8763, -5.5766) -> (-37.5267, -5.8469) projected
  line L568 (-37.5267, -5.8469) -> (-37.1977, -5.5796) projected
  line L569 (-37.1977, -9.0074) -> (-39.1423, -9.0074) projected
  line L570 (-37.1977, -11.4307) -> (-37.1977, -9.0074) projected
  line L571 (-37.1977, -9.0074) -> (-39.1423, -9.0074) projected
  line L572 (-39.1423, -9.0074) -> (-39.1423, -11.4307) projected
  line L573 (-39.1423, -11.4307) -> (-37.1977, -11.4307) projected
  line L574 (-37.2036, -16.5946) -> (-37.2036, -14.5238) projected
  line L575 (-37.7323, -14.5238) -> (-37.7323, -16.5916) projected
  line L576 (-37.7323, -16.5916) -> (-37.4533, -16.8325) projected
  line L577 (-37.4533, -16.8325) -> (-37.2036, -16.5946) projected
  line L578 (-38.6165, -16.5916) -> (-38.6165, -14.5238) projected
  line L579 (-38.6165, -14.5238) -> (-39.1423, -14.5238) projected
  line L580 (-39.1423, -14.5238) -> (-39.1423, -16.5946) projected
  line L581 (-39.1423, -16.5946) -> (-38.8926, -16.8325) projected
  line L582 (-38.8926, -16.8325) -> (-38.6165, -16.5916) projected
  line L583 (-37.1977, -22.4428) -> (-37.1977, -20.0195) projected
  line L584 (-37.1977, -20.0195) -> (-39.1423, -20.0195) projected
  line L585 (-39.1423, -20.0195) -> (-39.1423, -22.4428) projected
  line L586 (-39.1423, -22.4428) -> (-37.1977, -22.4428) projected
  line L587 (-37.1977, -34.3097) -> (-37.1977, -31.8864) projected
  line L588 (-39.1423, -34.3097) -> (-37.1977, -34.3097) projected
  line L589 (-39.1423, -31.8864) -> (-39.1423, -34.3097) projected
  line L590 (-37.1977, -31.8864) -> (-39.1423, -31.8864) projected
  line L591 (-39.2128, -35.5639) -> (-40.0969, -34.6798) projected
  line L592 (-37.1273, -35.5639) -> (-39.2128, -35.5639) projected
  line L593 (-36.2431, -34.6798) -> (-37.1273, -35.5639) projected
  line L594 (-36.2431, -31.5163) -> (-36.2431, -34.6798) projected
  line L595 (-37.1273, -30.6321) -> (-36.2431, -31.5163) projected
  line L596 (-39.2128, -30.6321) -> (-37.1273, -30.6321) projected
  line L597 (-40.0969, -31.5163) -> (-39.2128, -30.6321) projected
  line L598 (-40.0969, -34.6798) -> (-40.0969, -31.5163) projected
  line L599 (-37.1977, -34.3097) -> (-37.1977, -31.8864) projected
  line L600 (-37.1977, -31.8864) -> (-39.1423, -31.8864) projected
  line L601 (-39.1423, -31.8864) -> (-39.1423, -34.3097) projected
  line L602 (-39.1423, -34.3097) -> (-37.1977, -34.3097) projected
  line L603 (-63.6576, -44.1829) -> (-63.6576, -42.4249) projected
  line L604 (-74.1279, -38.9787) -> (-74.1279, -37.4229) projected
  line L605 (-74.1279, -37.4229) -> (-74.6556, -37.4229) projected
  line L606 (-74.6556, -37.4229) -> (-74.6556, -38.9787) projected
  line L607 (-74.6556, -38.9787) -> (-74.3861, -39.1798) projected
  line L608 (-74.3861, -39.1798) -> (-74.1279, -38.9787) projected
  line L609 (-74.1279, -16.7976) -> (-74.1279, -15.2418) projected
  line L610 (-74.1279, -16.7976) -> (-74.1279, -15.2418) projected
  line L611 (-74.1279, -15.2418) -> (-74.6556, -15.2418) projected
  line L612 (-74.6556, -15.2418) -> (-74.6556, -16.7976) projected
  line L613 (-74.6556, -16.7976) -> (-74.3861, -16.9986) projected
  line L614 (-74.3861, -16.9986) -> (-74.1279, -16.7976) projected
  line L615 (-63.4064, -0.2445) -> (-66.4201, -0.2445) projected
  line L616 (-66.4201, -0.2445) -> (-65.2101, -0.8039) projected
  line L617 (-65.2101, -0.8039) -> (-65.2101, -2.7331) projected
  line L618 (-65.2101, -2.7331) -> (-65.1644, -2.7331) projected
  line L619 (-57.5218, 15.0578) -> (-57.5218, 17.2347) projected
  line L620 (-57.5218, 17.2347) -> (-58.2757, 17.2347) projected
  line L621 (-58.2757, 17.2347) -> (-58.2757, 15.061) projected
  line L622 (-58.2757, 15.061) -> (-57.8873, 14.7771) projected
  line L623 (-57.8873, 14.7771) -> (-57.5218, 15.0578) projected
  line L624 (-59.0981, 9.2549) -> (-59.0981, 11.4318) projected
  line L625 (-59.0981, 11.4318) -> (-59.6823, 11.4318) projected
  line L626 (-59.6823, 11.4318) -> (-59.6823, 9.2516) projected
  line L627 (-59.6823, 9.2516) -> (-59.4049, 9.0036) projected
  line L628 (-59.4049, 9.0036) -> (-59.0981, 9.2549) projected
  line L629 (-57.5283, 9.2516) -> (-57.5283, 11.4318) projected
  line L630 (-57.5283, 11.4318) -> (-58.1125, 11.4318) projected
  line L631 (-58.1125, 11.4318) -> (-58.1125, 9.2549) projected
  line L632 (-58.1125, 9.2549) -> (-57.8057, 9.0036) projected
  line L633 (-57.8057, 9.0036) -> (-57.5283, 9.2516) projected
  line L634 (-57.5218, 3.08) -> (-57.5218, 5.6289) projected
  line L635 (-57.5218, 5.6289) -> (-59.6823, 5.6289) projected
  line L636 (-59.6823, 5.6289) -> (-59.6823, 3.08) projected
  line L637 (-59.6823, 3.08) -> (-57.5218, 3.08) projected
  line L638 (-51.9251, 17.2559) -> (-52.1356, 17.5248) projected
  line L639 (-52.0668, 17.0871) -> (-51.9251, 17.2559) projected
  line L640 (-52.2016, 16.9183) -> (-52.0668, 17.0871) projected
  line L641 (-52.2433, 17.0666) -> (-52.2016, 16.9183) projected
  line L642 (-52.2942, 17.1568) -> (-52.2433, 17.0666) projected
  line L643 (-52.3724, 17.2153) -> (-52.2942, 17.1568) projected
  line L644 (-52.4441, 17.2262) -> (-52.3724, 17.2153) projected
  line L645 (-52.4757, 17.1734) -> (-52.4441, 17.2262) projected
  line L646 (-52.4135, 16.995) -> (-52.4757, 17.1734) projected
  line L647 (-52.2703, 16.7263) -> (-52.4135, 16.995) projected
  line L648 (-52.1124, 16.4814) -> (-52.2703, 16.7263) projected
  line L649 (-52.0062, 16.3742) -> (-52.1124, 16.4814) projected
  line L650 (-51.9399, 16.3837) -> (-52.0062, 16.3742) projected
  line L651 (-51.9205, 16.4197) -> (-51.9399, 16.3837) projected
  line L652 (-52.0194, 16.6142) -> (-51.9205, 16.4197) projected
  line L653 (-52.0729, 16.7053) -> (-52.0194, 16.6142) projected
  line L654 (-52.0849, 16.7705) -> (-52.0729, 16.7053) projected
  line L655 (-51.9758, 16.9103) -> (-52.0849, 16.7705) projected
  line L656 (-51.8494, 16.9918) -> (-51.9758, 16.9103) projected
  line L657 (-51.8138, 16.9861) -> (-51.8494, 16.9918) projected
  line L658 (-51.7922, 16.9519) -> (-51.8138, 16.9861) projected
  line L659 (-51.7413, 16.8956) -> (-51.7922, 16.9519) projected
  line L660 (-51.6638, 16.8676) -> (-51.7413, 16.8956) projected
  line L661 (-51.5941, 16.8727) -> (-51.6638, 16.8676) projected
  line L662 (-51.5666, 16.9157) -> (-51.5941, 16.8727) projected
  line L663 (-51.7978, 17.3259) -> (-51.5666, 16.9157) projected
  line L664 (-51.9942, 17.6027) -> (-51.7978, 17.3259) projected
  line L665 (-52.1487, 17.7789) -> (-51.9942, 17.6027) projected
  line L666 (-52.2663, 17.8528) -> (-52.1487, 17.7789) projected
  line L667 (-52.2947, 17.8492) -> (-52.2663, 17.8528) projected
  line L668 (-52.3029, 17.8218) -> (-52.2947, 17.8492) projected
  line L669 (-52.2592, 17.7059) -> (-52.3029, 17.8218) projected
  line L670 (-52.1356, 17.5248) -> (-52.2592, 17.7059) projected
  line L671 (-52.782, 16.455) -> (-52.6361, 16.5567) projected
  line L672 (-52.8723, 16.3355) -> (-52.782, 16.455) projected
  line L673 (-52.8771, 16.2639) -> (-52.8723, 16.3355) projected
  line L674 (-52.8116, 16.2596) -> (-52.8771, 16.2639) projected
  line L675 (-52.6907, 16.3417) -> (-52.8116, 16.2596) projected
  line L676 (-52.5799, 16.4236) -> (-52.6907, 16.3417) projected
  line L677 (-52.5158, 16.4283) -> (-52.5799, 16.4236) projected
  line L678 (-52.5022, 16.3578) -> (-52.5158, 16.4283) projected
  line L679 (-52.5431, 16.2141) -> (-52.5022, 16.3578) projected
  line L680 (-52.5744, 16.0714) -> (-52.5431, 16.2141) projected
  line L681 (-52.5519, 15.9919) -> (-52.5744, 16.0714) projected
  line L682 (-52.4934, 15.9917) -> (-52.5519, 15.9919) projected
  line L683 (-52.4166, 16.0866) -> (-52.4934, 15.9917) projected
  line L684 (-52.3535, 16.2474) -> (-52.4166, 16.0866) projected
  line L685 (-52.3448, 16.3853) -> (-52.3535, 16.2474) projected
  line L686 (-52.3892, 16.4903) -> (-52.3448, 16.3853) projected
  line L687 (-52.4853, 16.5525) -> (-52.3892, 16.4903) projected
  line L688 (-52.6361, 16.5567) -> (-52.4853, 16.5525) projected
  line L689 (-52.8723, 16.3355) -> (-52.782, 16.455) projected
  line L690 (-52.782, 16.455) -> (-52.6361, 16.5567) projected
  line L691 (-52.6361, 16.5567) -> (-52.4853, 16.5525) projected
  line L692 (-52.4853, 16.5525) -> (-52.3892, 16.4903) projected
  line L693 (-52.3892, 16.4903) -> (-52.3448, 16.3853) projected
  line L694 (-52.3448, 16.3853) -> (-52.3535, 16.2474) projected
  line L695 (-52.3535, 16.2474) -> (-52.4166, 16.0866) projected
  line L696 (-52.4166, 16.0866) -> (-52.4934, 15.9917) projected
  line L697 (-52.4934, 15.9917) -> (-52.5519, 15.9919) projected
  line L698 (-52.5519, 15.9919) -> (-52.5744, 16.0714) projected
  line L699 (-52.5744, 16.0714) -> (-52.5431, 16.2141) projected
  line L700 (-52.5431, 16.2141) -> (-52.5022, 16.3578) projected
  line L701 (-52.5022, 16.3578) -> (-52.5158, 16.4283) projected
  line L702 (-52.5158, 16.4283) -> (-52.5799, 16.4236) projected
  line L703 (-52.5799, 16.4236) -> (-52.6907, 16.3417) projected
  line L704 (-52.6907, 16.3417) -> (-52.8116, 16.2596) projected
  line L705 (-52.8116, 16.2596) -> (-52.8771, 16.2639) projected
  line L706 (-52.8771, 16.2639) -> (-52.8723, 16.3355) projected
  line L707 (-53.2554, 15.5426) -> (-52.5089, 15.7104) projected
  line L708 (-52.5089, 15.7104) -> (-51.0336, 16.1022) projected
  line L709 (-51.0336, 16.1022) -> (-50.627, 16.2512) projected
  line L710 (-50.627, 16.2512) -> (-50.5157, 16.3102) projected
  line L711 (-50.5157, 16.3102) -> (-50.4619, 16.368) projected
  line L712 (-50.4619, 16.368) -> (-50.4627, 16.4313) projected
  line L713 (-50.4627, 16.4313) -> (-50.5151, 16.5069) projected
  line L714 (-50.5151, 16.5069) -> (-50.763, 16.722) projected
  line L715 (-50.763, 16.722) -> (-51.707, 17.5381) projected
  line L716 (-51.707, 17.5381) -> (-52.5133, 18.3589) projected
  line L717 (-52.5133, 18.3589) -> (-52.9595, 18.8264) projected
  line L718 (-52.9595, 18.8264) -> (-53.1528, 18.9965) projected
  line L719 (-53.1528, 18.9965) -> (-53.2683, 18.3468) projected
  line L720 (-53.2683, 18.3468) -> (-53.4283, 17.1675) projected
  line L721 (-53.4283, 17.1675) -> (-53.5616, 16.0265) projected
  line L722 (-53.5616, 16.0265) -> (-53.5973, 15.4916) projected
  line L723 (-53.5973, 15.4916) -> (-53.2554, 15.5426) projected
  line L724 (-52.0668, 17.0871) -> (-51.9251, 17.2559) projected
  line L725 (-51.9251, 17.2559) -> (-52.1356, 17.5248) projected
  line L726 (-52.1356, 17.5248) -> (-52.2592, 17.7059) projected
  line L727 (-52.2592, 17.7059) -> (-52.3029, 17.8218) projected
  line L728 (-52.3029, 17.8218) -> (-52.2947, 17.8492) projected
  line L729 (-52.2947, 17.8492) -> (-52.2663, 17.8528) projected
  line L730 (-52.2663, 17.8528) -> (-52.1487, 17.7789) projected
  line L731 (-52.1487, 17.7789) -> (-51.9942, 17.6027) projected
  line L732 (-51.9942, 17.6027) -> (-51.7978, 17.3259) projected
  line L733 (-51.7978, 17.3259) -> (-51.5666, 16.9157) projected
  line L734 (-51.5666, 16.9157) -> (-51.5941, 16.8727) projected
  line L735 (-51.5941, 16.8727) -> (-51.6638, 16.8676) projected
  line L736 (-51.6638, 16.8676) -> (-51.7413, 16.8956) projected
  line L737 (-51.7413, 16.8956) -> (-51.7922, 16.9519) projected
  line L738 (-51.7922, 16.9519) -> (-51.8138, 16.9861) projected
  line L739 (-51.8138, 16.9861) -> (-51.8494, 16.9918) projected
  line L740 (-51.8494, 16.9918) -> (-51.9758, 16.9103) projected
  line L741 (-51.9758, 16.9103) -> (-52.0849, 16.7705) projected
  line L742 (-52.0849, 16.7705) -> (-52.0729, 16.7053) projected
  line L743 (-52.0729, 16.7053) -> (-52.0194, 16.6142) projected
  line L744 (-52.0194, 16.6142) -> (-51.9205, 16.4197) projected
  line L745 (-51.9205, 16.4197) -> (-51.9399, 16.3837) projected
  line L746 (-51.9399, 16.3837) -> (-52.0062, 16.3742) projected
  line L747 (-52.0062, 16.3742) -> (-52.1124, 16.4814) projected
  line L748 (-52.1124, 16.4814) -> (-52.2703, 16.7263) projected
  line L749 (-52.2703, 16.7263) -> (-52.4135, 16.995) projected
  line L750 (-52.4135, 16.995) -> (-52.4757, 17.1734) projected
  line L751 (-52.4757, 17.1734) -> (-52.4441, 17.2262) projected
  line L752 (-52.4441, 17.2262) -> (-52.3724, 17.2153) projected
  line L753 (-52.3724, 17.2153) -> (-52.2942, 17.1568) projected
  line L754 (-52.2942, 17.1568) -> (-52.2433, 17.0666) projected
  line L755 (-52.2433, 17.0666) -> (-52.2016, 16.9183) projected
  line L756 (-52.2016, 16.9183) -> (-52.0668, 17.0871) projected
  line L757 (3.9927, -3.0535) -> (3.9927, -1.7806) projected
  line L758 (3.9927, -1.7806) -> (3.4111, -1.7806) projected
  line L759 (3.4111, -1.7806) -> (3.4111, -3.0535) projected
  line L760 (3.4111, -3.0535) -> (3.9927, -3.0535) projected
  line L761 (3.9927, -20.8537) -> (3.9927, -19.62) projected
  line L762 (3.9927, -19.62) -> (3.6441, -19.62) projected
  line L763 (3.6441, -19.62) -> (3.6441, -20.8518) projected
  line L764 (3.6441, -20.8518) -> (3.8282, -20.9947) projected
  line L765 (3.8282, -20.9947) -> (3.9927, -20.8537) projected
  line L766 (3.0527, -20.8518) -> (3.0527, -19.62) projected
  line L767 (3.0527, -19.62) -> (2.7042, -19.62) projected
  line L768 (2.7042, -19.62) -> (2.7042, -20.8537) projected
  line L769 (2.7042, -20.8537) -> (2.8686, -20.9947) projected
  line L770 (2.8686, -20.9947) -> (3.0527, -20.8518) projected
  line L771 (3.9985, -30.124) -> (3.9985, -28.6807) projected
  line L772 (3.9985, -28.6807) -> (2.7022, -28.6807) projected
  line L773 (2.7022, -28.6807) -> (2.7022, -30.124) projected
  line L774 (2.7022, -30.124) -> (3.9985, -30.124) projected
  line L775 (3.9985, -33.2199) -> (3.9985, -31.9882) projected
  line L776 (3.9985, -31.9882) -> (3.5462, -31.9882) projected
  line L777 (3.5462, -31.9882) -> (3.5462, -33.2199) projected
  line L778 (3.5462, -33.2199) -> (3.7792, -33.3805) projected
  line L779 (3.7792, -33.3805) -> (3.9985, -33.2199) projected
  line L780 (-54.9302, -67.3628) -> (-54.9302, -66.0372) projected
  line L781 (-53.0639, -66.0372) -> (-53.0639, -67.3628) projected
  line L782 (-56.647, -67.0289) -> (-56.647, -68.2) projected
  line L783 (-56.647, -68.2) -> (-57.1678, -68.2) projected
  line L784 (-57.1678, -68.2) -> (-57.1678, -65.2) projected
  line L785 (-57.1678, -65.2) -> (-56.3181, -65.2) projected
  line L786 (-56.3181, -67.0289) -> (-56.647, -67.0289) projected
  line L787 (-64.1968, -68.2) -> (-64.1968, -67.8088) projected
  line L788 (-64.1968, -67.8088) -> (-63.6387, -67.8088) projected
  line L789 (-63.6387, -67.8088) -> (-63.6387, -65.5912) projected
  line L790 (-63.6387, -65.5912) -> (-64.1968, -65.5912) projected
  line L791 (-64.1968, -65.5912) -> (-64.1968, -65.2) projected
  line L792 (-64.1968, -65.2) -> (-62.5548, -65.2) projected
  line L793 (-62.5548, -65.2) -> (-62.5548, -65.5912) projected
  line L794 (-62.5548, -65.5912) -> (-63.1129, -65.5912) projected
  line L795 (-76.0747, -68.2) -> (-76.0747, -65.2) projected
  line L796 (-76.0747, -65.2) -> (-75.5216, -65.2) projected
  line L797 (-75.5216, -65.2) -> (-75.098, -66.6726) projected
  line L798 (-75.098, -66.6726) -> (-74.6769, -65.2) projected
  line L799 (-74.6769, -65.2) -> (-74.1237, -65.2) projected
  line L800 (-74.1237, -65.2) -> (-74.1237, -68.2) projected
  line L801 (-74.1237, -68.2) -> (-74.6121, -68.2) projected
  line L802 (-74.6121, -68.2) -> (-74.6121, -67.5995) projected
  line L803 (-74.5274, -65.94) -> (-74.9211, -67.298) projected
  line L804 (-74.9211, -67.298) -> (-75.2774, -67.298) projected
  line L805 (-75.2774, -67.298) -> (-75.6711, -65.94) projected
  line L806 (-37.1273, -35.5639) -> (-39.2128, -35.5639) projected
  line L807 (-39.2128, -35.5639) -> (-40.0969, -34.6798) projected
  line L808 (-40.0969, -34.6798) -> (-40.0969, -31.5163) projected
  line L809 (-40.0969, -31.5163) -> (-39.2128, -30.6321) projected
  line L810 (-39.2128, -30.6321) -> (-37.1273, -30.6321) projected
  line L811 (-37.1273, -30.6321) -> (-36.2431, -31.5163) projected
  line L812 (-36.2431, -31.5163) -> (-36.2431, -34.6798) projected
  line L813 (-36.2431, -34.6798) -> (-37.1273, -35.5639) projected
  line L814 (-36.2431, -25.5358) -> (-40.0763, -25.5358) projected
  line L815 (-40.0763, -25.5358) -> (-40.7431, -24.2816) projected
  line L816 (-40.7431, -24.2816) -> (-36.2431, -24.2816) projected
  line L817 (-36.2431, -24.2816) -> (-36.2431, -25.5358) projected
  line L818 (-37.1273, -23.6971) -> (-39.2128, -23.6971) projected
  line L819 (-39.2128, -23.6971) -> (-40.0969, -22.8129) projected
  line L820 (-40.0969, -22.8129) -> (-40.0969, -19.6494) projected
  line L821 (-40.0969, -19.6494) -> (-39.2128, -18.7653) projected
  line L822 (-39.2128, -18.7653) -> (-37.1273, -18.7653) projected
  line L823 (-37.1273, -18.7653) -> (-36.2431, -19.6494) projected
  line L824 (-36.2431, -19.6494) -> (-36.2431, -22.8129) projected
  line L825 (-36.2431, -22.8129) -> (-37.1273, -23.6971) projected
  line L826 (4.635, -37.5613) -> (4.635, -40.3224) projected
  line L827 (4.635, -40.3224) -> (3.9927, -39.8015) projected
  line L828 (3.9927, -39.8015) -> (3.9927, -38.323) projected
  line L829 (3.9927, -38.323) -> (3.6441, -38.323) projected
  line L830 (3.6441, -38.323) -> (3.6441, -39.9973) projected
  line L831 (3.6441, -39.9973) -> (3.0527, -39.5176) projected
  line L832 (3.0527, -39.5176) -> (3.0527, -38.323) projected
  line L833 (3.0527, -38.323) -> (2.7042, -38.323) projected
  line L834 (2.7042, -38.323) -> (2.7042, -40.2441) projected
  line L835 (2.7042, -40.2441) -> (2.0619, -39.7193) projected
  line L836 (2.0619, -39.7193) -> (2.0619, -37.5613) projected
  line L837 (2.0619, -37.5613) -> (4.635, -37.5613) projected
  line L838 (4.635, -25.0404) -> (4.635, -27.8015) projected
  line L839 (4.635, -27.8015) -> (3.9927, -27.2806) projected
  line L840 (3.9927, -27.2806) -> (3.9927, -25.8022) projected
  line L841 (3.9927, -25.8022) -> (3.6421, -25.8022) projected
  line L842 (3.6421, -25.8022) -> (3.6421, -27.4764) projected
  line L843 (3.6421, -27.4764) -> (3.0508, -26.9967) projected
  line L844 (3.0508, -26.9967) -> (3.0508, -25.8022) projected
  line L845 (3.0508, -25.8022) -> (2.0795, -25.8022) projected
  line L846 (2.0795, -25.8022) -> (1.635, -25.0404) projected
  line L847 (1.635, -25.0404) -> (4.635, -25.0404) projected
  line L848 (3.8791, -22.7395) -> (3.2368, -22.7395) projected
  line L849 (3.2368, -22.7395) -> (3.2368, -22.1559) projected
  line L850 (3.2368, -22.1559) -> (3.8791, -22.1559) projected
  line L851 (3.8791, -22.1559) -> (3.8791, -22.7395) projected
  line L852 (5.0697, -18.5097) -> (2.6572, -18.5097) projected
  line L853 (2.6572, -18.5097) -> (2.0658, -17.9771) projected
  line L854 (2.0658, -17.9771) -> (2.0658, -16.2421) projected
  line L855 (2.0658, -16.2421) -> (2.6572, -15.7095) projected
  line L856 (2.6572, -15.7095) -> (4.6408, -15.7095) projected
  line L857 (2.7022, -16.4712) -> (2.7022, -17.7441) projected
  line L858 (2.7022, -17.7441) -> (4.6134, -17.7441) projected
  line L859 (4.6134, -17.7441) -> (5.0697, -18.5097) projected
  line L860 (4.635, -10.6279) -> (4.635, -12.8563) projected
  line L861 (2.7042, -12.778) -> (2.0619, -12.2532) projected
  line L862 (2.0619, -12.2532) -> (2.0619, -10.6259) projected
  line L863 (2.0619, -10.6259) -> (2.6454, -10.0952) projected
  line L864 (2.6454, -10.0952) -> (4.0416, -10.0952) projected
  line L865 (4.0416, -10.0952) -> (4.635, -10.6279) projected
  line L866 (2.7042, -4.949) -> (2.7042, -6.87) projected
  line L867 (2.7042, -6.87) -> (2.0619, -6.3452) projected
  line L868 (2.0619, -6.3452) -> (2.0619, -4.7179) projected
  line L869 (2.0619, -4.7179) -> (2.6454, -4.1873) projected
  line L870 (2.6454, -4.1873) -> (4.0416, -4.1873) projected
  line L871 (4.0514, -3.8191) -> (1.635, -3.8191) projected
  line L872 (1.635, -3.8191) -> (2.0795, -3.0535) projected
  line L873 (2.0795, -3.0535) -> (2.7786, -3.0535) projected
  line L874 (2.7786, -3.0535) -> (2.7786, -1.7806) projected
  line L875 (2.7786, -1.7806) -> (2.0619, -1.7806) projected
  line L876 (2.0619, -1.7806) -> (2.0658, -1.0189) projected